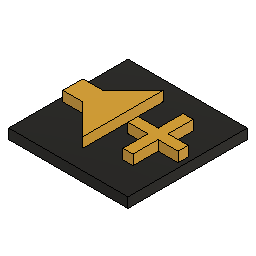
icon_volume (Autodesk Fusion 360 design; units mm, degrees)
Autodesk Fusion 360 part; units mm, degrees
sketch "Sketch1" plane through (0, 0, 0) normal (0, 0, 1) x (1, 0, 0)
  line L0 (5.95, -5.95) -> (-5.95, -5.95)
  line L1 (-5.95, -5.95) -> (-5.95, 5.95)
  line L2 (-5.95, 5.95) -> (5.95, 5.95)
  line L3 (5.95, 5.95) -> (5.95, -5.95)
  line L4 (5.95, -5.95) -> (-5.95, 5.95) construction
  line L5 (-5.95, -5.95) -> (5.95, 5.95) construction
  line L6 (-0.5, 3.5) -> (-0.5, 0)
  line L7 (0.5, 0) -> (0.5, 0.5)
  line L8 (2.5, 3) -> (3.5, 3)
  line L9 (5.5, 0.5) -> (5.5, -0.5)
  line L10 (3.5, -3) -> (2.5, -3)
  line L11 (0.5, 0) -> (0.5, -0.5)
  line L12 (0.5, 0.5) -> (2.5, 0.5)
  line L13 (2.5, 0.5) -> (2.5, 3)
  line L14 (3.5, 3) -> (3.5, 0.5)
  line L15 (3.5, 0.5) -> (5.5, 0.5)
  line L16 (5.5, -0.5) -> (3.5, -0.5)
  line L17 (3.5, -0.5) -> (3.5, -3)
  line L18 (2.5, -3) -> (2.5, -0.5)
  line L19 (2.5, -0.5) -> (0.5, -0.5)
  line L20 (-0.5, 0) -> (-0.5, -3.5)
  line L21 (-3.5, -1) -> (-5.5, -1)
  line L22 (-5.5, -1) -> (-5.5, 1)
  line L23 (-5.5, 1) -> (-3.5, 1)
  line L24 (-0.5, 3.5) -> (-0.5, 4)
  line L25 (-0.5, 4) -> (-3.5, 1)
  line L26 (-0.5, -3.5) -> (-0.5, -4)
  line L27 (-0.5, -4) -> (-3.5, -1)
  dimension "d1" = 11.9
  dimension "d2" = 11.9
  constraint horizontal L0
  constraint perpendicular L0 L1
  constraint parallel L0 L2
  constraint parallel L1 L3
  constraint coincident L4 origin
  constraint coincident L5 origin
  constraint parallel L1 L7
  constraint perpendicular L7 L12
  constraint perpendicular L8 L13
  constraint perpendicular L9 L15
  constraint perpendicular L9 L16
  constraint perpendicular L10 L17
  constraint perpendicular L10 L18
  constraint perpendicular L11 L19
  constraint parallel L6 L20
  constraint perpendicular L20 L21
  constraint perpendicular L21 L22
  constraint perpendicular L22 L23
  constraint parallel L6 L24
  constraint perpendicular L4 L25
  constraint parallel L24 L26
  constraint perpendicular L5 L27
  measures "d1" distance of L1.end L2.end
  measures "d2" distance of L0.end L1.end
extrude "Extrude1" add sketch "Sketch1" against normal blind 1 contours L0 L1 L2 L3 | L6 L20 L21 L22 L23 L24 L25 L26 L27 | L7 L8 L9 L10 L11 L12 L13 L14 L15 L16 L17 L18 L19
extrude "Extrude2" add sketch "Sketch1" along normal blind 1 contours L6 L20 L21 L22 L23 L24 L25 L26 L27 | L7 L8 L9 L10 L11 L12 L13 L14 L15 L16 L17 L18 L19
